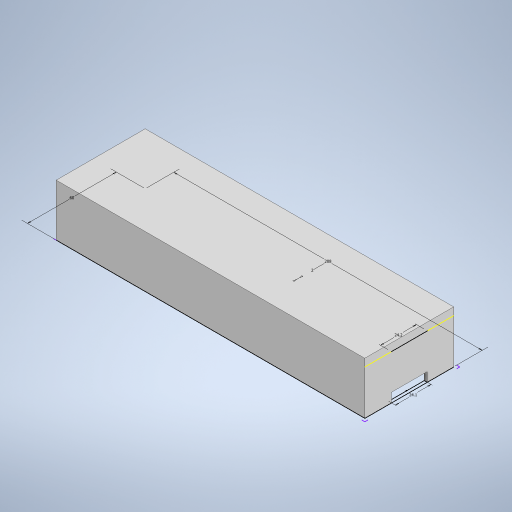
# Autodesk Inventor part: 막대바닥
Saved by Autodesk Inventor 2023 (Build 270158000, 158)
## iProperties
Created: 2023-04-29
Part Number: 막대바닥
Material: 일반
Document SubType Name: Modeling
Designer: rlatk
Density: 1 g/cm^3
Appearance: 기본값
Author: rlatk
Autodesk Inventor part; units mm, degrees
ref_plane "YZ Plane" through (0, 0, 0) normal (1, 0, 0) x (0, 1, 0)
ref_plane "XZ Plane" through (0, 0, 0) normal (0, 1, 0) x (-1, 0, 0)
ref_plane "XY Plane" through (0, 0, 0) normal (0, 0, 1) x (1, 0, 0)
sketch "스케치1" plane through (0, 0, 0) normal (0, 1, 0) x (-1, 0, 0)
  line L0 (0, 0) -> (208, 0)
  line L1 (208, 0) -> (208, -60)
  line L2 (208, -60) -> (0, -60)
  line L3 (0, -60) -> (0, 0)
  line L4 (-2, -62) -> (0, -62)
  line L5 (208, -62) -> (210, -62)
  line L6 (210, -62) -> (210, -60)
  line L7 (210, 0) -> (210, 0)
  line L8 (210, 0) -> (208, 0)
  line L9 (0, 2) -> (-2, 2)
  line L10 (-2, 2) -> (-2, 0)
  line L11 (-2, -60) -> (-2, -62)
  line L12 (2, -58) -> (206, -58)
  line L13 (206, -58) -> (206, -2)
  line L14 (206, -2) -> (2, -2)
  line L15 (2, -2) -> (2, -58)
  line L16 (2, -17.95) -> (2, -42.05)
  line L17 (2, -17.95) -> (0, -17.95)
  line L18 (2, -42.05) -> (0, -42.05)
  point P0 (2, -30)
  dimension "d0" = 208
  dimension "d1" = 60
  dimension "d3" = 2
  dimension "d9" = 24.1
  constraints: 38 end point, 13 parallel, 12 point on line, 6 perpendicular, 2 horizontal, 2 midpoint, 3 other
  measures "d0" distance of L1.end L2.end
  measures "d1" distance of L0.end L1.end
  measures "d3" distance between parallel lines of L2 L12
  measures "d9" distance of L16.start L16.end
extrude "돌출1" add sketch "스케치1" along normal blind 35
extrude "돌출2" cut sketch "스케치1" along normal blind 30 contours L15 L14 L13 L12
sketch "스케치2" plane through (0, 30, 0) normal (0, -1, 0) x (1, 0, 0)
  line L0 (-2, -2) -> (-2, -58) projected
  line L1 (-2, -17.9) -> (-2, -42.1)
  line L2 (-2, -17.9) -> (0, -17.9)
  line L3 (0, 0) -> (0, -60) projected
  line L4 (-2, -42.1) -> (0, -42.1)
  line L5 (0, -42.1) -> (0, -17.9)
  line L6 (0, -17.9) -> (0, -42.1)
  point P0 (-2, -30)
  dimension "d8" = 24.2
  constraints: 10 end point, 4 point on line, 2 equal length, 2 midpoint, 1 horizontal, 1 perpendicular
  measures "d8" distance of L1.start L1.end
extrude "돌출3" cut sketch "스케치1" along normal blind 6.1 contours L17 L15 L18 L3
